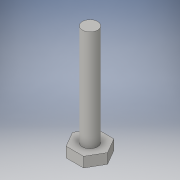
# Autodesk Inventor part: 3-8 2.5 Inch Hex Bolt
Saved by Autodesk Inventor 2016 (Build 200138000, 138)
## iProperties
Created: 2016-01-28
Part Number: 3-8 2.5 Inch Hex Bolt
Material: Generic
Document SubType Name: Modeling
Designer: Jack Jaworski
Density: 1 g/cm^3
Appearance: Default
Author: Jack Jaworski
Autodesk Inventor part; units mm, degrees
ref_plane "YZ Plane" through (0, 0, 0) normal (1, 0, 0) x (0, 1, 0)
ref_plane "XZ Plane" through (0, 0, 0) normal (0, 1, 0) x (-1, 0, 0)
ref_plane "XY Plane" through (0, 0, 0) normal (0, 0, 1) x (1, 0, 0)
sketch "Sketch1" plane through (0, 0, 0) normal (0, 1, 0) x (-1, 0, 0)
  line L0 (10.9985, 0) -> (5.4993, -9.525)
  line L1 (5.4993, -9.525) -> (-5.4993, -9.525)
  line L2 (-5.4993, -9.525) -> (-10.9985, 0)
  line L3 (-10.9985, 0) -> (-5.4993, 9.525)
  line L4 (-5.4993, 9.525) -> (5.4993, 9.525)
  line L5 (5.4993, 9.525) -> (10.9985, 0)
  point P0 (0, 0)
  point P1 (0, 0)
  dimension "d0" = 9.525
  constraints: 12 end point, 1 coincident, 1 horizontal, 13 other
  measures "d0" vertical distance of L0.start L0.end
extrude "Extrusion1" add sketch "Sketch1" along normal blind 6.35
sketch "Sketch2" plane through (0, 6.35, 0) normal (0, 1, 0) x (1, 0, 0)
  circle A0 centre (0, 0) radius 4.7625
  dimension "d3" = 9.525
  constraints: 1 centre point, 1 coincident
  measures "d3" diameter of A0
extrude "Extrusion2" add sketch "Sketch2" along normal blind 63.5
sketch "Sketch3" plane through (0, 0, 0) normal (0, -1, 0) x (1, 0, 0)
  point P0 (0, 0)
  point P1 (0, 0)
  constraints: 1 coincident
body "Solid1"
